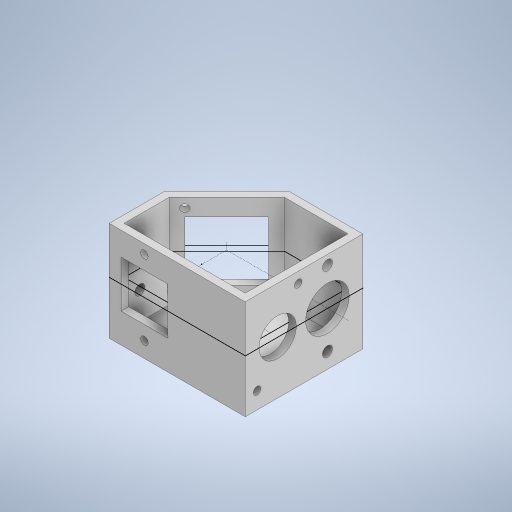
# Autodesk Inventor part: tactic2 chassis2
Saved by Autodesk Inventor 2024 (Build 280153000, 153)
## iProperties
Created: 2025-02-08
Part Number: tactic2 chassis2
Material: Generic
Document SubType Name: Modeling
Designer: Williamow
Density: 1 g/cm^3
Appearance: Default
Author: Williamow
Autodesk Inventor part; units mm, degrees
ref_plane "YZ Plane" through (0, 0, 0) normal (1, 0, 0) x (0, 1, 0)
ref_plane "XZ Plane" through (0, 0, 0) normal (0, 1, 0) x (-1, 0, 0)
ref_plane "XY Plane" through (0, 0, 0) normal (0, 0, 1) x (1, 0, 0)
sketch "Sketch1" plane through (0, 0, 0) normal (0, 1, 0) x (-1, 0, 0)
  line L0 (0, -4) -> (15, -4) construction
  line L1 (15, -4) -> (15, -12) construction
  line L2 (15, -12) -> (-4.6836, -12) construction
  line L3 (0, 0) -> (19.4569, 0)
  line L4 (19.4569, 0) -> (19.4569, -7.2603)
  line L5 (10.2172, -16.5) -> (0, -16.5)
  line L6 (0, -16.5) -> (0, 0)
  line L7 (-1.2, 1.2) -> (20.6569, 1.2)
  line L8 (20.6569, 1.2) -> (20.6569, -7.7574)
  line L9 (10.7142, -17.7) -> (-1.2, -17.7)
  line L10 (-1.2, -17.7) -> (-1.2, 1.2)
  line L11 (10.2172, -16.5) -> (19.4569, -7.2603)
  line L12 (20.6569, -7.7574) -> (10.7142, -17.7)
  line L13 (15, -12) -> (15.7071, -12.7071) construction
  line L14 (17.4749, -6.4749) -> (12.5251, -1.5251) construction
  line L15 (12.5251, -1.5251) -> (13.2676, -0.7827) construction
  line L16 (17.4749, -6.4749) -> (18.2173, -5.7324) construction
  line L17 (18.2173, -5.7324) -> (13.2676, -0.7827) construction
  line L18 (15, -12) -> (16.1863, -13.1863) construction
  point P0 (15, -8)
  dimension "d0" = 1.2
  dimension "d1" = 1.2
  dimension "d2" = 1.2
  dimension "d3" = 4
  dimension "d4" = 4.5
  dimension "d5" = 8
  dimension "d6" = 15
  dimension "d8" = 135
  dimension "d9" = 1.2
  dimension "d10" = 1.2
  dimension "d11" = 1
  dimension "d12" = 7
  dimension "d13" = 45
  dimension "d20" = 7
  dimension "d21" = 1.05
  dimension "d49" = 1.2395
  dimension "d68" = 4.4569
  dimension "d69" = 8
  constraints: 38 end point, 7 perpendicular, 6 parallel, 3 horizontal, 2 midpoint, 2 point on line
  measures "d0" distance between parallel lines of L6 L10
  measures "d1" distance between parallel lines of L7 L3
  measures "d2" distance between parallel lines of L9 L5
  measures "d3" distance between parallel lines of L3 L0
  measures "d4" distance between parallel lines of L5 L2
  measures "d5" distance of L0.end L1.end
  measures "d6" distance from line of L6 L1.end
  measures "d8" angle of L12 L8
  measures "d9" distance between parallel lines of L8 L4
  measures "d10" distance between parallel lines of L12 L11
  measures "d11" distance of L1.end L13.end
  measures "d12" distance of L8.end L13.end
  measures "d13" angle of L14 L1
  measures "d20" distance of L14.start L14.end
  measures "d21" distance of L14.end L15.end
  measures "d49" distance from line of L4 L16.end
  measures "d68" distance between parallel lines of L4 L1
  measures "d69" distance from line of L3 point (15, -8)
extrude "Extrusion1" add sketch "Sketch1" along normal mid plane 15
sketch "Sketch2" plane through (1.2, -7.5, -17.7) normal (1, 0, 0) x (0, 0, -1)
  circle A0 centre (-5.7, 7.5) radius 3.5
  circle A1 centre (-13.7, 7.5) radius 3
  circle A2 centre (-10.4, 13.3) radius 0.6
  circle A3 centre (-17, 1.7) radius 0.6
  line L0 (-10.4, 13.3) -> (-17, 1.7) construction
  line L1 (-16.7, 7.5) -> (-16.7, 7.5)
  circle A4 centre (-9.7, 1.5) radius 0.8
  line L2 (0, 0) -> (-18.9, 0) projected
  line L3 (-13.7, 7.5) -> (-5.7, 7.5) construction
  circle A5 centre (-5.7, 13.5) radius 0.8
  circle A6 centre (-5.7, 1.5) radius 0.8
  line L4 (-5.7, 1.5) -> (-5.7, 13.5) construction
  point P0 (-17.7, 7.5)
  point P1 (-5.7, 7.5)
  point P2 (-9.7, 7.5)
  dimension "d22" = 7
  dimension "d23" = 6
  dimension "d56" = 5.8
  dimension "d57" = 3.3
  dimension "d58" = 1.2
  dimension "d59" = 3
  dimension "d66" = 1.6
  dimension "d67" = 1.5
  dimension "d74" = 6
  constraints: 7 centre point, 6 end point, 3 coincident, 3 equal radius, 3 midpoint, 3 vertical alignment, 2 point on circle, 2 vertical
  measures "d22" diameter of A0
  measures "d23" diameter of A1
  measures "d56" vertical distance of L0.start point (-13.7, 7.5)
  measures "d57" horizontal distance of point (-13.7, 7.5) L0.start
  measures "d58" diameter of A2
  measures "d59" distance from line of A1.centre L1
  measures "d66" diameter of A4
  measures "d67" distance from line of L2 A4.centre
  measures "d74" distance of L4.end point (-5.7, 7.5)
extrude "Extrusion2" cut sketch "Sketch2" against normal blind 3 contours A0 | A1 | A2 | A3 | A5 | A6
sketch "Sketch3" plane through (-20.6569, -7.5, 1.2) normal (-1, 0, 0) x (0, 0, 1)
  circle A0 centre (-3.7, 10.5) radius 0.8
  circle A1 centre (-5.2, 7.5) radius 0.8 construction
  circle A2 centre (-3.7, 4.5) radius 0.8
  line L0 (-11.5, 6.75) -> (-11.5, 8.25)
  line L1 (-9.9, 6.75) -> (-9.9, 8.25)
  arc A3 (-9.9, 8.25) -> (-11.5, 8.25) centre (-10.7, 8.25) ccw
  arc A4 (-11.5, 6.75) -> (-9.9, 6.75) centre (-10.7, 6.75) ccw
  line L2 (-3.7, 4.5) -> (-3.7, 10.5) construction
  point P0 (-1.2, 7.5)
  point P1 (-5.2, 7.5)
  point P2 (-10.7, 7.5)
  point P3 (-11.5, 7.5)
  point P4 (-3.7, 7.5)
  dimension "d28" = 1.6
  dimension "d32" = 5.5
  dimension "d52" = 1.5
  dimension "d53" = 0.8
  dimension "d64" = 6
  dimension "d65" = 1.5
  constraints: 6 end point, 5 centre point, 4 point on circle, 4 tangent, 3 horizontal alignment, 3 vertical, 2 coincident, 2 equal radius, 2 midpoint, 2 vertical alignment
  measures "d28" diameter of A0
  measures "d32" distance of point (-10.7, 7.5) point (-5.2, 7.5)
  measures "d52" distance of L0.start L0.end
  measures "d53" radius of A4
  measures "d64" distance of L2.start L2.end
  measures "d65" distance from line of point (-5.2, 7.5) L2
extrude "Extrusion3" cut sketch "Sketch3" against normal blind 2 contours A0 | A2
sketch "Sketch4" plane through (-20.6569, -7.5, -7.7574) normal (-0.7071, 0, -0.7071) x (-0.7071, 0, 0.7071)
  line L0 (-11.75, 12.25) -> (-2.25, 12.25)
  line L1 (-2.25, 12.25) -> (-2.25, 2.75)
  line L2 (-2.25, 2.75) -> (-11.75, 2.75)
  line L3 (-11.75, 2.75) -> (-11.75, 12.25)
  circle A0 centre (-11.75, 13.5) radius 0.6
  circle A1 centre (-2.25, 13.5) radius 0.6
  circle A2 centre (-11.75, 1.5) radius 0.6
  circle A3 centre (-2.25, 1.5) radius 0.6
  point P0 (-9.1213, 7.5)
  point P1 (-7, 7.5)
  point P2 (-7, 7.5)
  point P3 (-7, 7.5)
  point P4 (-11.75, 7.5)
  point P5 (-7, 12.25)
  dimension "d35" = 9.5
  dimension "d36" = 6
  dimension "d37" = 6
  dimension "d38" = 1.2
  constraints: 8 end point, 5 vertical alignment, 4 centre point, 3 equal radius, 3 horizontal alignment, 2 midpoint, 2 parallel, 2 perpendicular, 1 horizontal
  measures "d35" distance of L0.start L0.end
  measures "d36" vertical distance of A0.centre point (-7, 7.5)
  measures "d37" vertical distance of A2.centre point (-7, 7.5)
  measures "d38" diameter of A1
extrude "Extrusion4" cut sketch "Sketch4" against normal blind 2 contours L0 L1 L2 L3 | A1 | A2
sketch "Sketch5" plane through (-20.6569, 7.5, 1.2) normal (0, 0, 1) x (1, 0, 0)
  line L0 (1.9069, -3.75) -> (9.4069, -3.75)
  line L1 (9.4069, -3.75) -> (9.4069, -11.25)
  line L2 (9.4069, -11.25) -> (1.9069, -11.25)
  line L3 (1.9069, -11.25) -> (1.9069, -3.75)
  circle A0 centre (5.6569, -1.5) radius 0.6
  circle A1 centre (5.6569, -13.5) radius 0.6
  arc A2 (13.6569, -12.7) -> (13.6569, -14.3) centre (13.6569, -13.5) ccw
  arc A3 (17.6569, -14.3) -> (17.6569, -12.7) centre (17.6569, -13.5) ccw
  line L4 (13.6569, -12.7) -> (17.6569, -12.7)
  line L5 (13.6569, -14.3) -> (17.6569, -14.3)
  point P0 (20.6569, -7.5)
  point P1 (5.6569, -7.5)
  point P2 (5.6569, -7.5)
  point P3 (5.6569, -7.5)
  point P4 (9.4069, -7.5)
  point P5 (5.6569, -3.75)
  point P6 (15.6569, -12.7)
  dimension "d41" = 7.5
  dimension "d42" = 6
  dimension "d43" = 6
  dimension "d44" = 1.2
  dimension "d70" = 1.6
  dimension "d71" = 6
  dimension "d72" = 10
  dimension "d73" = 4
  constraints: 12 end point, 4 centre point, 4 point on circle, 4 tangent, 3 midpoint, 3 parallel, 3 vertical alignment, 2 horizontal, 2 perpendicular, 1 equal radius, 1 horizontal alignment
  measures "d41" distance of L0.start L0.end
  measures "d42" distance of A0.centre point (5.657, -7.5)
  measures "d43" distance of A1.centre point (5.657, -7.5)
  measures "d44" diameter of A0
  measures "d70" distance between parallel lines of L4 L5
  measures "d71" vertical distance of point (5.657, -7.5) A2.centre
  measures "d72" horizontal distance of point (15.657, -12.7) point (5.657, -7.5)
  measures "d73" distance of L4.start L4.end
extrude "Extrusion5" cut sketch "Sketch5" against normal blind 2 contours L0 L1 L2 L3 | A0 | A1
sketch "Sketch6" plane through (0, -7.5, 0) normal (0, -1, 0) x (1, 0, 0)
  line L0 (1.2, -17.7) -> (1.2, 1.2) projected
  line L1 (1.2, 1.2) -> (-20.6569, 1.2) projected
  line L2 (-20.6569, 1.2) -> (-20.6569, -7.7574) projected
  line L3 (-20.6569, -7.7574) -> (-10.7142, -17.7) projected
  line L4 (-10.7142, -17.7) -> (1.2, -17.7) projected
  line L5 (-15, -4) -> (-15, -12) construction
  line L6 (1.2, -10.187) -> (1.2, -11.787) projected
  circle A0 centre (-15, -8) radius 0.8
  circle A1 centre (-10, -8) radius 0.8
  point P0 (0, 0)
  dimension "d61" = 1.6
  dimension "d62" = 5
  constraints: 2 centre point, 2 coincident, 1 equal radius, 1 horizontal alignment, 1 midpoint
  measures "d61" diameter of A0
  measures "d62" distance of A0.centre A1.centre
extrude "Extrusion6" add sketch "Sketch6" along normal blind 1 contours L4 L3 L2 L1 L0 | A0
body "Solid1"
